Autodesk Fusion 360 part; units mm, degrees
(part 2 of 3)
sketch "Sketch22" plane through (0, -42.5, 42.5) normal (0, -0.707107, 0.707107) x (1, 0, 0) in component "BOX"
  line L0 (10.5, 0.9066) -> (16.8, 0.9066)
  line L1 (16.8, 0.9066) -> (16.8, -5.3934)
  line L2 (16.8, -5.3934) -> (10.5, -5.3934)
  line L3 (10.5, -5.3934) -> (10.5, -4.8934)
  line L4 (10.5, -4.8934) -> (16.5, -4.8934)
  line L5 (16.5, -4.8934) -> (16.5, 0.4066)
  line L6 (16.5, 0.4066) -> (10.5, 0.4066)
  line L7 (10.5, 0.4066) -> (10.5, 0.9066)
  line L8 (33.8, 0.9066) -> (40.1, 0.9066)
  line L9 (40.1, 0.9066) -> (40.1, -5.3934)
  line L10 (40.1, -5.3934) -> (33.8, -5.3934)
  line L11 (33.8, -5.3934) -> (33.8, -4.8934)
  line L12 (33.8, -4.8934) -> (39.8, -4.8934)
  line L13 (39.8, -4.8934) -> (39.8, 0.4066)
  line L14 (39.8, 0.4066) -> (33.8, 0.4066)
  line L15 (33.8, 0.4066) -> (33.8, 0.9066)
  line L16 (44.1, 0.9066) -> (50.4, 0.9066)
  line L17 (50.4, 0.9066) -> (50.4, -5.3934)
  line L18 (50.4, -5.3934) -> (44.1, -5.3934)
  line L19 (44.1, -5.3934) -> (44.1, -4.8934)
  line L20 (44.1, -4.8934) -> (50.1, -4.8934)
  line L21 (50.1, -4.8934) -> (50.1, 0.4066)
  line L22 (50.1, 0.4066) -> (44.1, 0.4066)
  line L23 (44.1, 0.4066) -> (44.1, 0.9066)
  line L24 (20.8, 0.9066) -> (27.1, 0.9066)
  line L25 (27.1, 0.9066) -> (27.1, -5.3934)
  line L26 (27.1, -5.3934) -> (20.8, -5.3934)
  line L27 (20.8, -5.3934) -> (20.8, -4.8934)
  line L28 (20.8, -4.8934) -> (26.8, -4.8934)
  line L29 (26.8, -4.8934) -> (26.8, 0.4066)
  line L30 (26.8, 0.4066) -> (20.8, 0.4066)
  line L31 (20.8, 0.4066) -> (20.8, 0.9066)
  line L32 (-10.3, 0.9066) -> (-4, 0.9066)
  line L33 (-4, 0.9066) -> (-4, -5.3934)
  line L34 (-4, -5.3934) -> (-10.3, -5.3934)
  line L35 (-10.3, -5.3934) -> (-10.3, -4.8934)
  line L36 (-10.3, -4.8934) -> (-4.3, -4.8934)
  line L37 (-4.3, -4.8934) -> (-4.3, 0.4066)
  line L38 (-4.3, 0.4066) -> (-10.3, 0.4066)
  line L39 (-10.3, 0.4066) -> (-10.3, 0.9066)
  line L40 (-54.5, -15.7434) -> (-54.5, 7.2566)
  line L41 (-54.5, 7.2566) -> (-20, 7.2566)
  line L42 (-20, 7.2566) -> (-20, -15.7434)
  line L43 (-20, -15.7434) -> (-54.5, -15.7434)
  line L44 (65, -24.7487) -> (65, 17.6777)
  line L45 (65, 17.6777) -> (-65, 17.6777)
  line L46 (-65, 17.6777) -> (-65, -24.7487)
  line L47 (-65, -24.7487) -> (65, -24.7487)
  line L48 (-10.546, -7.6932) -> (-10.2963, -7.6713)
  spline S0 degree 2 poles (-10.2963, -7.6713) (-10.2786, -7.8214) (-10.2138, -7.9176) knots 0 0 0 1 1 1
  spline S1 degree 2 poles (-10.2138, -7.9176) (-10.149, -8.0138) (-10.0125, -8.0731) knots 0 0 0 1 1 1
  spline S2 degree 2 poles (-10.0125, -8.0731) (-9.8761, -8.1325) (-9.7056, -8.1325) knots 0 0 0 1 1 1
  spline S3 degree 2 poles (-9.7056, -8.1325) (-9.5541, -8.1325) (-9.4382, -8.0874) knots 0 0 0 1 1 1
  spline S4 degree 2 poles (-9.4382, -8.0874) (-9.3222, -8.0424) (-9.2656, -7.964) knots 0 0 0 1 1 1
  spline S5 degree 2 poles (-9.2656, -7.964) (-9.209, -7.8855) (-9.209, -7.7928) knots 0 0 0 1 1 1
  spline S6 degree 2 poles (-9.209, -7.7928) (-9.209, -7.6986) (-9.2636, -7.6284) knots 0 0 0 1 1 1
  spline S7 degree 2 poles (-9.2636, -7.6284) (-9.3181, -7.5581) (-9.4436, -7.5104) knots 0 0 0 1 1 1
  spline S8 degree 2 poles (-9.4436, -7.5104) (-9.5241, -7.479) (-9.7997, -7.4128) knots 0 0 0 1 1 1
  spline S9 degree 2 poles (-9.7997, -7.4128) (-10.0753, -7.3467) (-10.1858, -7.288) knots 0 0 0 1 1 1
  spline S10 degree 2 poles (-10.1858, -7.288) (-10.329, -7.213) (-10.3993, -7.1018) knots 0 0 0 1 1 1
  spline S11 degree 2 poles (-10.3993, -7.1018) (-10.4696, -6.9906) (-10.4696, -6.8528) knots 0 0 0 1 1 1
  spline S12 degree 2 poles (-10.4696, -6.8528) (-10.4696, -6.7014) (-10.3836, -6.5697) knots 0 0 0 1 1 1
  spline S13 degree 2 poles (-10.3836, -6.5697) (-10.2977, -6.4381) (-10.1326, -6.3698) knots 0 0 0 1 1 1
  spline S14 degree 2 poles (-10.1326, -6.3698) (-9.9675, -6.3016) (-9.7656, -6.3016) knots 0 0 0 1 1 1
  spline S15 degree 2 poles (-9.7656, -6.3016) (-9.5432, -6.3016) (-9.3734, -6.3733) knots 0 0 0 1 1 1
  spline S16 degree 2 poles (-9.3734, -6.3733) (-9.2035, -6.4449) (-9.1121, -6.584) knots 0 0 0 1 1 1
  spline S17 degree 2 poles (-9.1121, -6.584) (-9.0207, -6.7232) (-9.0139, -6.8992) knots 0 0 0 1 1 1
  line L49 (-9.0139, -6.8992) -> (-9.2676, -6.9183)
  spline S18 degree 2 poles (-9.2676, -6.9183) (-9.2881, -6.7286) (-9.4061, -6.6318) knots 0 0 0 1 1 1
  spline S19 degree 2 poles (-9.4061, -6.6318) (-9.5241, -6.5349) (-9.7547, -6.5349) knots 0 0 0 1 1 1
  spline S20 degree 2 poles (-9.7547, -6.5349) (-9.9948, -6.5349) (-10.1046, -6.6229) knots 0 0 0 1 1 1
  spline S21 degree 2 poles (-10.1046, -6.6229) (-10.2144, -6.7109) (-10.2144, -6.8351) knots 0 0 0 1 1 1
  spline S22 degree 2 poles (-10.2144, -6.8351) (-10.2144, -6.9428) (-10.1367, -7.0124) knots 0 0 0 1 1 1
  spline S23 degree 2 poles (-10.1367, -7.0124) (-10.0603, -7.082) (-9.7376, -7.155) knots 0 0 0 1 1 1
  spline S24 degree 2 poles (-9.7376, -7.155) (-9.415, -7.228) (-9.2949, -7.2825) knots 0 0 0 1 1 1
  spline S25 degree 2 poles (-9.2949, -7.2825) (-9.1203, -7.363) (-9.0371, -7.4865) knots 0 0 0 1 1 1
  spline S26 degree 2 poles (-9.0371, -7.4865) (-8.9539, -7.61) (-8.9539, -7.7709) knots 0 0 0 1 1 1
  spline S27 degree 2 poles (-8.9539, -7.7709) (-8.9539, -7.9306) (-9.0453, -8.0718) knots 0 0 0 1 1 1
  spline S28 degree 2 poles (-9.0453, -8.0718) (-9.1367, -8.213) (-9.3079, -8.2914) knots 0 0 0 1 1 1
  spline S29 degree 2 poles (-9.3079, -8.2914) (-9.4791, -8.3698) (-9.6933, -8.3698) knots 0 0 0 1 1 1
  spline S30 degree 2 poles (-9.6933, -8.3698) (-9.9648, -8.3698) (-10.1483, -8.2907) knots 0 0 0 1 1 1
  spline S31 degree 2 poles (-10.1483, -8.2907) (-10.3318, -8.2116) (-10.4361, -8.0527) knots 0 0 0 1 1 1
  spline S32 degree 2 poles (-10.4361, -8.0527) (-10.5405, -7.8937) (-10.546, -7.6932) knots 0 0 0 1 1 1
  line L50 (-8.0835, -8.3357) -> (-8.0835, -6.5718)
  line L51 (-8.0835, -6.5718) -> (-8.7424, -6.5718)
  line L52 (-8.7424, -6.5718) -> (-8.7424, -6.3357)
  line L53 (-8.7424, -6.3357) -> (-7.1571, -6.3357)
  line L54 (-7.1571, -6.3357) -> (-7.1571, -6.5718)
  line L55 (-7.1571, -6.5718) -> (-7.8188, -6.5718)
  line L56 (-7.8188, -6.5718) -> (-7.8188, -8.3357)
  line L57 (-7.8188, -8.3357) -> (-8.0835, -8.3357)
  line L58 (-7.3127, -8.3357) -> (-6.5446, -6.3357)
  line L59 (-6.5446, -6.3357) -> (-6.2595, -6.3357)
  line L60 (-6.2595, -6.3357) -> (-5.4409, -8.3357)
  line L61 (-5.4409, -8.3357) -> (-5.7424, -8.3357)
  line L62 (-5.7424, -8.3357) -> (-5.9757, -7.73)
  line L63 (-5.9757, -7.73) -> (-6.812, -7.73)
  line L64 (-6.812, -7.73) -> (-7.0316, -8.3357)
  line L65 (-7.0316, -8.3357) -> (-7.3127, -8.3357)
  line L66 (-6.7356, -7.5145) -> (-6.0575, -7.5145)
  line L67 (-6.0575, -7.5145) -> (-6.2663, -6.9606)
  spline S33 degree 2 poles (-6.2663, -6.9606) (-6.3618, -6.7082) (-6.4082, -6.5458) knots 0 0 0 1 1 1
  spline S34 degree 2 poles (-6.4082, -6.5458) (-6.4464, -6.7382) (-6.5159, -6.9278) knots 0 0 0 1 1 1
  line L68 (-6.5159, -6.9278) -> (-6.7356, -7.5145)
  line L69 (-5.2254, -8.3357) -> (-5.2254, -6.3357)
  line L70 (-5.2254, -6.3357) -> (-4.3386, -6.3357)
  spline S35 degree 2 poles (-4.3386, -6.3357) (-4.0712, -6.3357) (-3.932, -6.3896) knots 0 0 0 1 1 1
  spline S36 degree 2 poles (-3.932, -6.3896) (-3.7929, -6.4435) (-3.7097, -6.5799) knots 0 0 0 1 1 1
  spline S37 degree 2 poles (-3.7097, -6.5799) (-3.6264, -6.7164) (-3.6264, -6.8814) knots 0 0 0 1 1 1
  spline S38 degree 2 poles (-3.6264, -6.8814) (-3.6264, -7.0943) (-3.7642, -7.2402) knots 0 0 0 1 1 1
  spline S39 degree 2 poles (-3.7642, -7.2402) (-3.902, -7.3862) (-4.1899, -7.4258) knots 0 0 0 1 1 1
  spline S40 degree 2 poles (-4.1899, -7.4258) (-4.0848, -7.4763) (-4.0303, -7.5254) knots 0 0 0 1 1 1
  spline S41 degree 2 poles (-4.0303, -7.5254) (-3.9143, -7.6318) (-3.8106, -7.7914) knots 0 0 0 1 1 1
  line L71 (-3.8106, -7.7914) -> (-3.4627, -8.3357)
  line L72 (-3.4627, -8.3357) -> (-3.7956, -8.3357)
  line L73 (-3.7956, -8.3357) -> (-4.0603, -7.9196)
  spline S42 degree 2 poles (-4.0603, -7.9196) (-4.1762, -7.7396) (-4.2513, -7.6441) knots 0 0 0 1 1 1
  spline S43 degree 2 poles (-4.2513, -7.6441) (-4.3263, -7.5486) (-4.3857, -7.5104) knots 0 0 0 1 1 1
  spline S44 degree 2 poles (-4.3857, -7.5104) (-4.445, -7.4722) (-4.5064, -7.4572) knots 0 0 0 1 1 1
  spline S45 degree 2 poles (-4.5064, -7.4572) (-4.5514, -7.4476) (-4.6537, -7.4476) knots 0 0 0 1 1 1
  line L74 (-4.6537, -7.4476) -> (-4.9607, -7.4476)
  line L75 (-4.9607, -7.4476) -> (-4.9607, -8.3357)
  line L76 (-4.9607, -8.3357) -> (-5.2254, -8.3357)
  line L77 (-4.9607, -7.2184) -> (-4.3918, -7.2184)
  spline S46 degree 2 poles (-4.3918, -7.2184) (-4.2103, -7.2184) (-4.108, -7.1809) knots 0 0 0 1 1 1
  spline S47 degree 2 poles (-4.108, -7.1809) (-4.0057, -7.1434) (-3.9525, -7.0608) knots 0 0 0 1 1 1
  spline S48 degree 2 poles (-3.9525, -7.0608) (-3.8993, -6.9783) (-3.8993, -6.8814) knots 0 0 0 1 1 1
  spline S49 degree 2 poles (-3.8993, -6.8814) (-3.8993, -6.7396) (-4.0023, -6.6482) knots 0 0 0 1 1 1
  spline S50 degree 2 poles (-4.0023, -6.6482) (-4.1053, -6.5567) (-4.3277, -6.5567) knots 0 0 0 1 1 1
  line L78 (-4.3277, -6.5567) -> (-4.9607, -6.5567)
  line L79 (-4.9607, -6.5567) -> (-4.9607, -7.2184)
  line L80 (-2.7533, -8.3357) -> (-2.7533, -6.5718)
  line L81 (-2.7533, -6.5718) -> (-3.4123, -6.5718)
  line L82 (-3.4123, -6.5718) -> (-3.4123, -6.3357)
  line L83 (-3.4123, -6.3357) -> (-1.827, -6.3357)
  line L84 (-1.827, -6.3357) -> (-1.827, -6.5718)
  line L85 (-1.827, -6.5718) -> (-2.4887, -6.5718)
  line L86 (-2.4887, -6.5718) -> (-2.4887, -8.3357)
  line L87 (-2.4887, -8.3357) -> (-2.7533, -8.3357)
  line L88 (-9.7656, -6.3016) -> (65, -6.3016) construction
  line L89 (10.1816, -8.2989) -> (10.1816, -6.2989)
  line L90 (10.1816, -6.2989) -> (10.58, -6.2989)
  line L91 (10.58, -6.2989) -> (11.0533, -7.715)
  spline S51 degree 2 poles (11.0533, -7.715) (11.1188, -7.9129) (11.1488, -8.0111) knots 0 0 0 1 1 1
  spline S52 degree 2 poles (11.1488, -8.0111) (11.183, -7.9019) (11.2553, -7.6905) knots 0 0 0 1 1 1
  line L92 (11.2553, -7.6905) -> (11.7341, -6.2989)
  line L93 (11.7341, -6.2989) -> (12.0902, -6.2989)
  line L94 (12.0902, -6.2989) -> (12.0902, -8.2989)
  line L95 (12.0902, -8.2989) -> (11.8351, -8.2989)
  line L96 (11.8351, -8.2989) -> (11.8351, -6.625)
  line L97 (11.8351, -6.625) -> (11.2539, -8.2989)
  line L98 (11.2539, -8.2989) -> (11.0151, -8.2989)
  line L99 (11.0151, -8.2989) -> (10.4367, -6.5963)
  line L100 (10.4367, -6.5963) -> (10.4367, -8.2989)
  line L101 (10.4367, -8.2989) -> (10.1816, -8.2989)
  line L102 (12.5227, -8.2989) -> (12.5227, -6.2989)
  line L103 (12.5227, -6.2989) -> (13.9688, -6.2989)
  line L104 (13.9688, -6.2989) -> (13.9688, -6.535)
  line L105 (13.9688, -6.535) -> (12.7873, -6.535)
  line L106 (12.7873, -6.535) -> (12.7873, -7.1475)
  line L107 (12.7873, -7.1475) -> (13.8937, -7.1475)
  line L108 (13.8937, -7.1475) -> (13.8937, -7.3822)
  line L109 (13.8937, -7.3822) -> (12.7873, -7.3822)
  line L110 (12.7873, -7.3822) -> (12.7873, -8.0629)
  line L111 (12.7873, -8.0629) -> (14.0151, -8.0629)
  line L112 (14.0151, -8.0629) -> (14.0151, -8.2989)
  line L113 (14.0151, -8.2989) -> (12.5227, -8.2989)
  line L114 (14.378, -8.2989) -> (14.378, -6.2989)
  line L115 (14.378, -6.2989) -> (14.6495, -6.2989)
  line L116 (14.6495, -6.2989) -> (15.7, -7.8692)
  line L117 (15.7, -7.8692) -> (15.7, -6.2989)
  line L118 (15.7, -6.2989) -> (15.9538, -6.2989)
  line L119 (15.9538, -6.2989) -> (15.9538, -8.2989)
  line L120 (15.9538, -8.2989) -> (15.6823, -8.2989)
  line L121 (15.6823, -8.2989) -> (14.6318, -6.7273)
  line L122 (14.6318, -6.7273) -> (14.6318, -8.2989)
  line L123 (14.6318, -8.2989) -> (14.378, -8.2989)
  line L124 (17.7109, -6.2989) -> (17.9756, -6.2989)
  line L125 (17.9756, -6.2989) -> (17.9756, -7.4545)
  spline S53 degree 2 poles (17.9756, -7.4545) (17.9756, -7.756) (17.9074, -7.9333) knots 0 0 0 1 1 1
  spline S54 degree 2 poles (17.9074, -7.9333) (17.8392, -8.1107) (17.6611, -8.2219) knots 0 0 0 1 1 1
  spline S55 degree 2 poles (17.6611, -8.2219) (17.4831, -8.333) (17.1939, -8.333) knots 0 0 0 1 1 1
  spline S56 degree 2 poles (17.1939, -8.333) (16.9128, -8.333) (16.7341, -8.2362) knots 0 0 0 1 1 1
  spline S57 degree 2 poles (16.7341, -8.2362) (16.5554, -8.1393) (16.479, -7.9558) knots 0 0 0 1 1 1
  spline S58 degree 2 poles (16.479, -7.9558) (16.4026, -7.7723) (16.4026, -7.4545) knots 0 0 0 1 1 1
  line L126 (16.4026, -7.4545) -> (16.4026, -6.2989)
  line L127 (16.4026, -6.2989) -> (16.6673, -6.2989)
  line L128 (16.6673, -6.2989) -> (16.6673, -7.4531)
  spline S59 degree 2 poles (16.6673, -7.4531) (16.6673, -7.7137) (16.7157, -7.8371) knots 0 0 0 1 1 1
  spline S60 degree 2 poles (16.7157, -7.8371) (16.7641, -7.9606) (16.8821, -8.0274) knots 0 0 0 1 1 1
  spline S61 degree 2 poles (16.8821, -8.0274) (17.0001, -8.0943) (17.1707, -8.0943) knots 0 0 0 1 1 1
  spline S62 degree 2 poles (17.1707, -8.0943) (17.4626, -8.0943) (17.5868, -7.962) knots 0 0 0 1 1 1
  spline S63 degree 2 poles (17.5868, -7.962) (17.7109, -7.8296) (17.7109, -7.4531) knots 0 0 0 1 1 1
  line L129 (17.7109, -7.4531) -> (17.7109, -6.2989)
  line L130 (20.4857, -7.8167) -> (20.7354, -7.7948)
  spline S64 degree 2 poles (20.7354, -7.7948) (20.7531, -7.9449) (20.8179, -8.0411) knots 0 0 0 1 1 1
  spline S65 degree 2 poles (20.8179, -8.0411) (20.8827, -8.1373) (21.0191, -8.1966) knots 0 0 0 1 1 1
  spline S66 degree 2 poles (21.0191, -8.1966) (21.1556, -8.256) (21.3261, -8.256) knots 0 0 0 1 1 1
  spline S67 degree 2 poles (21.3261, -8.256) (21.4775, -8.256) (21.5935, -8.2109) knots 0 0 0 1 1 1
  spline S68 degree 2 poles (21.5935, -8.2109) (21.7094, -8.1659) (21.7661, -8.0875) knots 0 0 0 1 1 1
  spline S69 degree 2 poles (21.7661, -8.0875) (21.8227, -8.009) (21.8227, -7.9163) knots 0 0 0 1 1 1
  spline S70 degree 2 poles (21.8227, -7.9163) (21.8227, -7.8221) (21.7681, -7.7519) knots 0 0 0 1 1 1
  spline S71 degree 2 poles (21.7681, -7.7519) (21.7135, -7.6816) (21.588, -7.6339) knots 0 0 0 1 1 1
  spline S72 degree 2 poles (21.588, -7.6339) (21.5075, -7.6025) (21.2319, -7.5363) knots 0 0 0 1 1 1
  spline S73 degree 2 poles (21.2319, -7.5363) (20.9564, -7.4701) (20.8459, -7.4115) knots 0 0 0 1 1 1
  spline S74 degree 2 poles (20.8459, -7.4115) (20.7026, -7.3364) (20.6324, -7.2253) knots 0 0 0 1 1 1
  spline S75 degree 2 poles (20.6324, -7.2253) (20.5621, -7.1141) (20.5621, -6.9763) knots 0 0 0 1 1 1
  spline S76 degree 2 poles (20.5621, -6.9763) (20.5621, -6.8248) (20.648, -6.6932) knots 0 0 0 1 1 1
  spline S77 degree 2 poles (20.648, -6.6932) (20.734, -6.5615) (20.8991, -6.4933) knots 0 0 0 1 1 1
  spline S78 degree 2 poles (20.8991, -6.4933) (21.0641, -6.4251) (21.2661, -6.4251) knots 0 0 0 1 1 1
  spline S79 degree 2 poles (21.2661, -6.4251) (21.4884, -6.4251) (21.6583, -6.4967) knots 0 0 0 1 1 1
  spline S80 degree 2 poles (21.6583, -6.4967) (21.8281, -6.5684) (21.9195, -6.7075) knots 0 0 0 1 1 1
  spline S81 degree 2 poles (21.9195, -6.7075) (22.0109, -6.8467) (22.0178, -7.0227) knots 0 0 0 1 1 1
  line L131 (22.0178, -7.0227) -> (21.764, -7.0418)
  spline S82 degree 2 poles (21.764, -7.0418) (21.7435, -6.8521) (21.6255, -6.7553) knots 0 0 0 1 1 1
  spline S83 degree 2 poles (21.6255, -6.7553) (21.5075, -6.6584) (21.277, -6.6584) knots 0 0 0 1 1 1
  spline S84 degree 2 poles (21.277, -6.6584) (21.0369, -6.6584) (20.927, -6.7464) knots 0 0 0 1 1 1
  spline S85 degree 2 poles (20.927, -6.7464) (20.8172, -6.8344) (20.8172, -6.9585) knots 0 0 0 1 1 1
  spline S86 degree 2 poles (20.8172, -6.9585) (20.8172, -7.0663) (20.895, -7.1359) knots 0 0 0 1 1 1
  spline S87 degree 2 poles (20.895, -7.1359) (20.9714, -7.2055) (21.294, -7.2785) knots 0 0 0 1 1 1
  spline S88 degree 2 poles (21.294, -7.2785) (21.6167, -7.3514) (21.7367, -7.406) knots 0 0 0 1 1 1
  spline S89 degree 2 poles (21.7367, -7.406) (21.9113, -7.4865) (21.9946, -7.61) knots 0 0 0 1 1 1
  spline S90 degree 2 poles (21.9946, -7.61) (22.0778, -7.7334) (22.0778, -7.8944) knots 0 0 0 1 1 1
  spline S91 degree 2 poles (22.0778, -7.8944) (22.0778, -8.054) (21.9864, -8.1952) knots 0 0 0 1 1 1
  spline S92 degree 2 poles (21.9864, -8.1952) (21.895, -8.3364) (21.7238, -8.4149) knots 0 0 0 1 1 1
  spline S93 degree 2 poles (21.7238, -8.4149) (21.5525, -8.4933) (21.3384, -8.4933) knots 0 0 0 1 1 1
  spline S94 degree 2 poles (21.3384, -8.4933) (21.0669, -8.4933) (20.8834, -8.4142) knots 0 0 0 1 1 1
  spline S95 degree 2 poles (20.8834, -8.4142) (20.6999, -8.3351) (20.5955, -8.1761) knots 0 0 0 1 1 1
  spline S96 degree 2 poles (20.5955, -8.1761) (20.4912, -8.0172) (20.4857, -7.8167) knots 0 0 0 1 1 1
  line L132 (22.4448, -8.4592) -> (22.4448, -6.4592)
  line L133 (22.4448, -6.4592) -> (23.8909, -6.4592)
  line L134 (23.8909, -6.4592) -> (23.8909, -6.6952)
  line L135 (23.8909, -6.6952) -> (22.7094, -6.6952)
  line L136 (22.7094, -6.6952) -> (22.7094, -7.3078)
  line L137 (22.7094, -7.3078) -> (23.8159, -7.3078)
  line L138 (23.8159, -7.3078) -> (23.8159, -7.5424)
  line L139 (23.8159, -7.5424) -> (22.7094, -7.5424)
  line L140 (22.7094, -7.5424) -> (22.7094, -8.2232)
  line L141 (22.7094, -8.2232) -> (23.9373, -8.2232)
  line L142 (23.9373, -8.2232) -> (23.9373, -8.4592)
  line L143 (23.9373, -8.4592) -> (22.4448, -8.4592)
  line L144 (24.292, -8.4592) -> (24.292, -6.4592)
  line L145 (24.292, -6.4592) -> (24.5566, -6.4592)
  line L146 (24.5566, -6.4592) -> (24.5566, -8.2232)
  line L147 (24.5566, -8.2232) -> (25.5416, -8.2232)
  line L148 (25.5416, -8.2232) -> (25.5416, -8.4592)
  line L149 (25.5416, -8.4592) -> (24.292, -8.4592)
  line L150 (25.8622, -8.4592) -> (25.8622, -6.4592)
  line L151 (25.8622, -6.4592) -> (27.3083, -6.4592)
  line L152 (27.3083, -6.4592) -> (27.3083, -6.6952)
  line L153 (27.3083, -6.6952) -> (26.1269, -6.6952)
  line L154 (26.1269, -6.6952) -> (26.1269, -7.3078)
  line L155 (26.1269, -7.3078) -> (27.2333, -7.3078)
  line L156 (27.2333, -7.3078) -> (27.2333, -7.5424)
  line L157 (27.2333, -7.5424) -> (26.1269, -7.5424)
  line L158 (26.1269, -7.5424) -> (26.1269, -8.2232)
  line L159 (26.1269, -8.2232) -> (27.3547, -8.2232)
  line L160 (27.3547, -8.2232) -> (27.3547, -8.4592)
  line L161 (27.3547, -8.4592) -> (25.8622, -8.4592)
  line L162 (29.1474, -7.758) -> (29.412, -7.8248)
  spline S97 degree 2 poles (29.412, -7.8248) (29.3288, -8.1509) (29.1126, -8.3221) knots 0 0 0 1 1 1
  spline S98 degree 2 poles (29.1126, -8.3221) (28.8963, -8.4933) (28.5839, -8.4933) knots 0 0 0 1 1 1
  spline S99 degree 2 poles (28.5839, -8.4933) (28.2606, -8.4933) (28.058, -8.3617) knots 0 0 0 1 1 1
  spline S100 degree 2 poles (28.058, -8.3617) (27.8554, -8.23) (27.7497, -7.9804) knots 0 0 0 1 1 1
  spline S101 degree 2 poles (27.7497, -7.9804) (27.644, -7.7307) (27.644, -7.4442) knots 0 0 0 1 1 1
  spline S102 degree 2 poles (27.644, -7.4442) (27.644, -7.1318) (27.7633, -6.8992) knots 0 0 0 1 1 1
  spline S103 degree 2 poles (27.7633, -6.8992) (27.8827, -6.6666) (28.103, -6.5459) knots 0 0 0 1 1 1
  spline S104 degree 2 poles (28.103, -6.5459) (28.3234, -6.4251) (28.588, -6.4251) knots 0 0 0 1 1 1
  spline S105 degree 2 poles (28.588, -6.4251) (28.8882, -6.4251) (29.0928, -6.5779) knots 0 0 0 1 1 1
  spline S106 degree 2 poles (29.0928, -6.5779) (29.2974, -6.7307) (29.3779, -7.0077) knots 0 0 0 1 1 1
  line L163 (29.3779, -7.0077) -> (29.1174, -7.069)
  spline S107 degree 2 poles (29.1174, -7.069) (29.0478, -6.8508) (28.9154, -6.7512) knots 0 0 0 1 1 1
  spline S108 degree 2 poles (28.9154, -6.7512) (28.7831, -6.6516) (28.5826, -6.6516) knots 0 0 0 1 1 1
  spline S109 degree 2 poles (28.5826, -6.6516) (28.352, -6.6516) (28.1972, -6.7621) knots 0 0 0 1 1 1
  spline S110 degree 2 poles (28.1972, -6.7621) (28.0423, -6.8726) (27.9796, -7.0588) knots 0 0 0 1 1 1
  spline S111 degree 2 poles (27.9796, -7.0588) (27.9168, -7.245) (27.9168, -7.4429) knots 0 0 0 1 1 1
  spline S112 degree 2 poles (27.9168, -7.4429) (27.9168, -7.698) (27.9912, -7.8883) knots 0 0 0 1 1 1
  spline S113 degree 2 poles (27.9912, -7.8883) (28.0655, -8.0786) (28.2224, -8.1727) knots 0 0 0 1 1 1
  spline S114 degree 2 poles (28.2224, -8.1727) (28.3793, -8.2669) (28.5621, -8.2669) knots 0 0 0 1 1 1
  spline S115 degree 2 poles (28.5621, -8.2669) (28.7845, -8.2669) (28.9386, -8.1386) knots 0 0 0 1 1 1
  spline S116 degree 2 poles (28.9386, -8.1386) (29.0928, -8.0104) (29.1474, -7.758) knots 0 0 0 1 1 1
  line L164 (30.247, -8.4592) -> (30.247, -6.6952)
  line L165 (30.247, -6.6952) -> (29.588, -6.6952)
  line L166 (29.588, -6.6952) -> (29.588, -6.4592)
  line L167 (29.588, -6.4592) -> (31.1733, -6.4592)
  line L168 (31.1733, -6.4592) -> (31.1733, -6.6952)
  line L169 (31.1733, -6.6952) -> (30.5116, -6.6952)
  line L170 (30.5116, -6.6952) -> (30.5116, -8.4592)
  line L171 (30.5116, -8.4592) -> (30.247, -8.4592)
  line L172 (36.1107, -6.5124) -> (36.3754, -6.5124)
  line L173 (36.3754, -6.5124) -> (36.3754, -7.668)
  spline S117 degree 2 poles (36.3754, -7.668) (36.3754, -7.9695) (36.3072, -8.1468) knots 0 0 0 1 1 1
  spline S118 degree 2 poles (36.3072, -8.1468) (36.2389, -8.3242) (36.0609, -8.4354) knots 0 0 0 1 1 1
  spline S119 degree 2 poles (36.0609, -8.4354) (35.8829, -8.5465) (35.5936, -8.5465) knots 0 0 0 1 1 1
  spline S120 degree 2 poles (35.5936, -8.5465) (35.3126, -8.5465) (35.1339, -8.4497) knots 0 0 0 1 1 1
  spline S121 degree 2 poles (35.1339, -8.4497) (34.9552, -8.3528) (34.8788, -8.1693) knots 0 0 0 1 1 1
  spline S122 degree 2 poles (34.8788, -8.1693) (34.8024, -7.9858) (34.8024, -7.668) knots 0 0 0 1 1 1
  line L174 (34.8024, -7.668) -> (34.8024, -6.5124)
  line L175 (34.8024, -6.5124) -> (35.067, -6.5124)
  line L176 (35.067, -6.5124) -> (35.067, -7.6666)
  spline S123 degree 2 poles (35.067, -7.6666) (35.067, -7.9272) (35.1155, -8.0506) knots 0 0 0 1 1 1
  spline S124 degree 2 poles (35.1155, -8.0506) (35.1639, -8.1741) (35.2819, -8.2409) knots 0 0 0 1 1 1
  spline S125 degree 2 poles (35.2819, -8.2409) (35.3999, -8.3078) (35.5705, -8.3078) knots 0 0 0 1 1 1
  spline S126 degree 2 poles (35.5705, -8.3078) (35.8624, -8.3078) (35.9866, -8.1755) knots 0 0 0 1 1 1
  spline S127 degree 2 poles (35.9866, -8.1755) (36.1107, -8.0431) (36.1107, -7.6666) knots 0 0 0 1 1 1
  line L177 (36.1107, -7.6666) -> (36.1107, -6.5124)
  line L178 (36.816, -8.5124) -> (36.816, -6.5124)
  line L179 (36.816, -6.5124) -> (37.5705, -6.5124)
  spline S128 degree 2 poles (37.5705, -6.5124) (37.7696, -6.5124) (37.8747, -6.5315) knots 0 0 0 1 1 1
  spline S129 degree 2 poles (37.8747, -6.5315) (38.022, -6.5561) (38.1216, -6.625) knots 0 0 0 1 1 1
  spline S130 degree 2 poles (38.1216, -6.625) (38.2212, -6.6939) (38.2819, -6.818) knots 0 0 0 1 1 1
  spline S131 degree 2 poles (38.2819, -6.818) (38.3426, -6.9422) (38.3426, -7.0909) knots 0 0 0 1 1 1
  spline S132 degree 2 poles (38.3426, -7.0909) (38.3426, -7.346) (38.1803, -7.5227) knots 0 0 0 1 1 1
  spline S133 degree 2 poles (38.1803, -7.5227) (38.0179, -7.6993) (37.5936, -7.6993) knots 0 0 0 1 1 1
  line L180 (37.5936, -7.6993) -> (37.0807, -7.6993)
  line L181 (37.0807, -7.6993) -> (37.0807, -8.5124)
  line L182 (37.0807, -8.5124) -> (36.816, -8.5124)
  line L183 (37.0807, -7.4633) -> (37.5977, -7.4633)
  spline S134 degree 2 poles (37.5977, -7.4633) (37.8542, -7.4633) (37.962, -7.3678) knots 0 0 0 1 1 1
  spline S135 degree 2 poles (37.962, -7.3678) (38.0698, -7.2723) (38.0698, -7.0991) knots 0 0 0 1 1 1
  spline S136 degree 2 poles (38.0698, -7.0991) (38.0698, -6.9736) (38.0063, -6.8842) knots 0 0 0 1 1 1
  spline S137 degree 2 poles (38.0063, -6.8842) (37.9429, -6.7948) (37.8392, -6.7662) knots 0 0 0 1 1 1
  spline S138 degree 2 poles (37.8392, -6.7662) (37.7724, -6.7485) (37.5923, -6.7485) knots 0 0 0 1 1 1
  line L184 (37.5923, -6.7485) -> (37.0807, -6.7485)
  line L185 (37.0807, -6.7485) -> (37.0807, -7.4633)
  line L186 (38.464, -8.5465) -> (39.0439, -6.4783)
  line L187 (39.0439, -6.4783) -> (39.2403, -6.4783)
  line L188 (39.2403, -6.4783) -> (38.6619, -8.5465)
  line L189 (38.6619, -8.5465) -> (38.464, -8.5465)
  line L190 (39.9402, -8.1891) -> (39.9402, -7.6407)
  line L191 (39.9402, -7.6407) -> (39.3958, -7.6407)
  line L192 (39.3958, -7.6407) -> (39.3958, -7.4115)
  line L193 (39.3958, -7.4115) -> (39.9402, -7.4115)
  line L194 (39.9402, -7.4115) -> (39.9402, -6.8671)
  line L195 (39.9402, -6.8671) -> (40.1721, -6.8671)
  line L196 (40.1721, -6.8671) -> (40.1721, -7.4115)
  line L197 (40.1721, -7.4115) -> (40.7164, -7.4115)
  line L198 (40.7164, -7.4115) -> (40.7164, -7.6407)
  line L199 (40.7164, -7.6407) -> (40.1721, -7.6407)
  line L200 (40.1721, -7.6407) -> (40.1721, -8.1891)
  line L201 (40.1721, -8.1891) -> (39.9402, -8.1891)
  line L202 (43.102, -8.34) -> (43.102, -6.34)
  line L203 (43.102, -6.34) -> (43.7909, -6.34)
  spline S139 degree 2 poles (43.7909, -6.34) (44.0242, -6.34) (44.147, -6.3686) knots 0 0 0 1 1 1
  spline S140 degree 2 poles (44.147, -6.3686) (44.3189, -6.4082) (44.4403, -6.5119) knots 0 0 0 1 1 1
  spline S141 degree 2 poles (44.4403, -6.5119) (44.5985, -6.6456) (44.677, -6.8536) knots 0 0 0 1 1 1
  spline S142 degree 2 poles (44.677, -6.8536) (44.7554, -7.0617) (44.7554, -7.3291) knots 0 0 0 1 1 1
  spline S143 degree 2 poles (44.7554, -7.3291) (44.7554, -7.5569) (44.7022, -7.7329) knots 0 0 0 1 1 1
  spline S144 degree 2 poles (44.7022, -7.7329) (44.649, -7.9089) (44.5658, -8.0242) knots 0 0 0 1 1 1
  spline S145 degree 2 poles (44.5658, -8.0242) (44.4826, -8.1394) (44.3837, -8.2056) knots 0 0 0 1 1 1
  spline S146 degree 2 poles (44.3837, -8.2056) (44.2848, -8.2718) (44.1449, -8.3059) knots 0 0 0 1 1 1
  spline S147 degree 2 poles (44.1449, -8.3059) (44.0051, -8.34) (43.8237, -8.34) knots 0 0 0 1 1 1
  line L204 (43.8237, -8.34) -> (43.102, -8.34)
  line L205 (43.3666, -8.104) -> (43.7936, -8.104)
  spline S148 degree 2 poles (43.7936, -8.104) (43.9915, -8.104) (44.104, -8.0671) knots 0 0 0 1 1 1
  spline S149 degree 2 poles (44.104, -8.0671) (44.2166, -8.0303) (44.2834, -7.9635) knots 0 0 0 1 1 1
  spline S150 degree 2 poles (44.2834, -7.9635) (44.3775, -7.8693) (44.4301, -7.7104) knots 0 0 0 1 1 1
  spline S151 degree 2 poles (44.4301, -7.7104) (44.4826, -7.5515) (44.4826, -7.325) knots 0 0 0 1 1 1
  spline S152 degree 2 poles (44.4826, -7.325) (44.4826, -7.0112) (44.3796, -6.8427) knots 0 0 0 1 1 1
  spline S153 degree 2 poles (44.3796, -6.8427) (44.2766, -6.6742) (44.1292, -6.6169) knots 0 0 0 1 1 1
  spline S154 degree 2 poles (44.1292, -6.6169) (44.0228, -6.576) (43.7868, -6.576) knots 0 0 0 1 1 1
  line L206 (43.7868, -6.576) -> (43.3666, -6.576)
  line L207 (43.3666, -6.576) -> (43.3666, -8.104)
  spline S155 degree 2 poles (45.0392, -7.3659) (45.0392, -6.868) (45.3066, -6.5862) knots 0 0 0 1 1 1
  spline S156 degree 2 poles (45.3066, -6.5862) (45.574, -6.3045) (45.9969, -6.3045) knots 0 0 0 1 1 1
  spline S157 degree 2 poles (45.9969, -6.3045) (46.2739, -6.3045) (46.4962, -6.4369) knots 0 0 0 1 1 1
  spline S158 degree 2 poles (46.4962, -6.4369) (46.7186, -6.5692) (46.8352, -6.8059) knots 0 0 0 1 1 1
  spline S159 degree 2 poles (46.8352, -6.8059) (46.9519, -7.0426) (46.9519, -7.3427) knots 0 0 0 1 1 1
  spline S160 degree 2 poles (46.9519, -7.3427) (46.9519, -7.6469) (46.8291, -7.8871) knots 0 0 0 1 1 1
  spline S161 degree 2 poles (46.8291, -7.8871) (46.7063, -8.1272) (46.4812, -8.2506) knots 0 0 0 1 1 1
  spline S162 degree 2 poles (46.4812, -8.2506) (46.2561, -8.3741) (45.9955, -8.3741) knots 0 0 0 1 1 1
  spline S163 degree 2 poles (45.9955, -8.3741) (45.7131, -8.3741) (45.4908, -8.2377) knots 0 0 0 1 1 1
  spline S164 degree 2 poles (45.4908, -8.2377) (45.2684, -8.1012) (45.1538, -7.8652) knots 0 0 0 1 1 1
  spline S165 degree 2 poles (45.1538, -7.8652) (45.0392, -7.6292) (45.0392, -7.3659) knots 0 0 0 1 1 1
  spline S166 degree 2 poles (45.3121, -7.37) (45.3121, -7.7315) (45.5065, -7.9396) knots 0 0 0 1 1 1
  spline S167 degree 2 poles (45.5065, -7.9396) (45.7009, -8.1476) (45.9942, -8.1476) knots 0 0 0 1 1 1
  spline S168 degree 2 poles (45.9942, -8.1476) (46.293, -8.1476) (46.486, -7.9375) knots 0 0 0 1 1 1
  spline S169 degree 2 poles (46.486, -7.9375) (46.679, -7.7274) (46.679, -7.3414) knots 0 0 0 1 1 1
  spline S170 degree 2 poles (46.679, -7.3414) (46.679, -7.0972) (46.5965, -6.915) knots 0 0 0 1 1 1
  spline S171 degree 2 poles (46.5965, -6.915) (46.514, -6.7329) (46.355, -6.6326) knots 0 0 0 1 1 1
  spline S172 degree 2 poles (46.355, -6.6326) (46.1961, -6.5324) (45.9983, -6.5324) knots 0 0 0 1 1 1
  spline S173 degree 2 poles (45.9983, -6.5324) (45.7172, -6.5324) (45.5146, -6.7254) knots 0 0 0 1 1 1
  spline S174 degree 2 poles (45.5146, -6.7254) (45.3121, -6.9184) (45.3121, -7.37) knots 0 0 0 1 1 1
  line L208 (47.6422, -8.34) -> (47.1115, -6.34)
  line L209 (47.1115, -6.34) -> (47.383, -6.34)
  line L210 (47.383, -6.34) -> (47.6872, -7.651)
  spline S175 degree 2 poles (47.6872, -7.651) (47.7363, -7.857) (47.7718, -8.0603) knots 0 0 0 1 1 1
  spline S176 degree 2 poles (47.7718, -8.0603) (47.8482, -7.7397) (47.8618, -7.6906) knots 0 0 0 1 1 1
  line L211 (47.8618, -7.6906) -> (48.2425, -6.34)
  line L212 (48.2425, -6.34) -> (48.5617, -6.34)
  line L213 (48.5617, -6.34) -> (48.8482, -7.3523)
  spline S177 degree 2 poles (48.8482, -7.3523) (48.956, -7.7288) (49.0037, -8.0603) knots 0 0 0 1 1 1
  spline S178 degree 2 poles (49.0037, -8.0603) (49.0419, -7.8707) (49.1033, -7.6251) knots 0 0 0 1 1 1
  line L214 (49.1033, -7.6251) -> (49.4171, -6.34)
  line L215 (49.4171, -6.34) -> (49.6831, -6.34)
  line L216 (49.6831, -6.34) -> (49.1347, -8.34)
  line L217 (49.1347, -8.34) -> (48.8796, -8.34)
  line L218 (48.8796, -8.34) -> (48.458, -6.8161)
  spline S179 degree 2 poles (48.458, -6.8161) (48.4048, -6.6251) (48.3953, -6.5815) knots 0 0 0 1 1 1
  spline S180 degree 2 poles (48.3953, -6.5815) (48.3639, -6.7193) (48.3366, -6.8161) knots 0 0 0 1 1 1
  line L219 (48.3366, -6.8161) -> (47.9123, -8.34)
  line L220 (47.9123, -8.34) -> (47.6422, -8.34)
  line L221 (49.9273, -8.34) -> (49.9273, -6.34)
  line L222 (49.9273, -6.34) -> (50.1988, -6.34)
  line L223 (50.1988, -6.34) -> (51.2493, -7.9102)
  line L224 (51.2493, -7.9102) -> (51.2493, -6.34)
  line L225 (51.2493, -6.34) -> (51.503, -6.34)
  line L226 (51.503, -6.34) -> (51.503, -8.34)
  line L227 (51.503, -8.34) -> (51.2316, -8.34)
  line L228 (51.2316, -8.34) -> (50.1811, -6.7684)
  line L229 (50.1811, -6.7684) -> (50.1811, -8.34)
  line L230 (50.1811, -8.34) -> (49.9273, -8.34)
  line L231 (51.7322, -8.3741) -> (52.3121, -6.3059)
  line L232 (52.3121, -6.3059) -> (52.5085, -6.3059)
  line L233 (52.5085, -6.3059) -> (51.9301, -8.3741)
  line L234 (51.9301, -8.3741) -> (51.7322, -8.3741)
  line L235 (52.5972, -7.7397) -> (52.5972, -7.4928)
  line L236 (52.5972, -7.4928) -> (53.3516, -7.4928)
  line L237 (53.3516, -7.4928) -> (53.3516, -7.7397)
  line L238 (53.3516, -7.7397) -> (52.5972, -7.7397)
  constraint coincident L44 L88.end
extrude "Extrude23" cut sketch "Sketch22" against normal blind 3 contours L48 S0 S1 S2 S3 S4 S5 S6 S7 S8 S9 S10 S11 S12 S13 S14 S15 S16 S17 L49 S18 S19 S20 S21 S22 S23 S24 S25 S26 S27 S28 S29 S30 S31 S32 | L50 L51 L52 L53 L54 L55 L56 L57 | L58 L59 L60 L61 L62 L63 L64 L65 | L69 L70 S35 S36 S37 S38 S39 S40 S41 L71 L72 L73 S42 S43 S44 S45 L74 L75 L76 | L80 L81 L82 L83 L84 L85 L86 L87 | L89 L90 L91 S51 S52 L92 L93 L94 L95 L96 L97 L98 L99 L100 L101 | L102 L103 L104 L105 L106 L107 L108 L109 L110 L111 L112 L113 | L114 L115 L116 L117 L118 L119 L120 L121 L122 L123 | L124 L125 S53 S54 S55 S56 S57 S58 L126 L127 L128 S59 S60 S61 S62 S63 L129 | L130 S64 S65 S66 S67 S68 S69 S70 S71 S72 S73 S74 S75 S76 S77 S78 S79 S80 S81 L131 S82 S83 S84 S85 S86 S87 S88 S89 S90 S91 S92 S93 S94 S95 S96 | L132 L133 L134 L135 L136 L137 L138 L139 L140 L141 L142 L143 | L144 L145 L146 L147 L148 L149 | L150 L151 L152 L153 L154 L155 L156 L157 L158 L159 L160 L161 | L162 S97 S98 S99 S100 S101 S102 S103 S104 S105 S106 L163 S107 S108 S109 S110 S111 S112 S113 S114 S115 S116 | L164 L165 L166 L167 L168 L169 L170 L171 | L172 L173 S117 S118 S119 S120 S121 S122 L174 L175 L176 S123 S124 S125 S126 S127 L177 | L178 L179 S128 S129 S130 S131 S132 S133 L180 L181 L182 | L186 L187 L188 L189 | L190 L191 L192 L193 L194 L195 L196 L197 L198 L199 L200 L201 | L202 L203 S139 S140 S141 S142 S143 S144 S145 S146 S147 L204 | S155 S156 S157 S158 S159 S160 S161 S162 S163 S164 S165 | L208 L209 L210 S175 S176 L211 L212 L213 S177 S178 L214 L215 L216 L217 L218 S179 S180 L219 L220 | L221 L222 L223 L224 L225 L226 L227 L228 L229 L230 | L231 L232 L233 L234 | L235 L236 L237 L238 bodies 2 makes body 4 at (45.3177, -46.5494, 36.3293) makes body 5 at (37.0807, -46.0262, 36.1454) makes body 6 at (-4.9607, -45.8781, 36.2935) makes body 7 at (43.3666, -47.1631, 36.4227) makes body 8 at (-6.5096, -46.3993, 35.7723) in component "BOX"
sketch "Sketch23" plane through (0, 0, 55) normal (0, 0, 1) x (-1, 0, 0) in component "BOX"
  line L0 (65, 30) -> (-65, 30)
  line L1 (-65, 30) -> (-65, -60)
  line L2 (-65, -60) -> (65, -60)
  line L3 (65, -60) -> (65, 30)
  line L4 (56.8223, 1.6907) -> (56.8223, -8.0112)
  line L5 (56.8223, -8.0112) -> (60.4465, -8.0112)
  line L6 (60.4465, -8.0112) -> (60.4465, -9.3093)
  line L7 (60.4465, -9.3093) -> (51.7275, -9.3093)
  line L8 (51.7275, -9.3093) -> (51.7275, -8.0112)
  line L9 (51.7275, -8.0112) -> (55.3667, -8.0112)
  line L10 (55.3667, -8.0112) -> (55.3667, 1.6907)
  line L11 (55.3667, 1.6907) -> (56.8223, 1.6907)
  line L12 (50.2043, 1.6907) -> (50.2043, -9.3093)
  line L13 (50.2043, -9.3093) -> (42.2507, -9.3093)
  line L14 (42.2507, -9.3093) -> (42.2507, -8.0112)
  line L15 (42.2507, -8.0112) -> (48.7487, -8.0112)
  line L16 (48.7487, -8.0112) -> (48.7487, -4.6422)
  line L17 (48.7487, -4.6422) -> (42.6634, -4.6422)
  line L18 (42.6634, -4.6422) -> (42.6634, -3.3516)
  line L19 (42.6634, -3.3516) -> (48.7487, -3.3516)
  line L20 (48.7487, -3.3516) -> (48.7487, 0.3926)
  line L21 (48.7487, 0.3926) -> (41.9956, 0.3926)
  line L22 (41.9956, 0.3926) -> (41.9956, 1.6907)
  line L23 (41.9956, 1.6907) -> (50.2043, 1.6907)
  line L24 (32.1361, -2.1661) -> (30.6805, -1.7984)
  spline S0 degree 2 poles (30.6805, -1.7984) (31.1382, -0.0051) (32.3275, 0.9366) knots 0 0 0 1 1 1
  spline S1 degree 2 poles (32.3275, 0.9366) (33.5167, 1.8783) (35.235, 1.8783) knots 0 0 0 1 1 1
  spline S2 degree 2 poles (35.235, 1.8783) (37.0133, 1.8783) (38.1276, 1.1542) knots 0 0 0 1 1 1
  spline S3 degree 2 poles (38.1276, 1.1542) (39.2418, 0.4301) (39.8234, -0.943) knots 0 0 0 1 1 1
  spline S4 degree 2 poles (39.8234, -0.943) (40.4049, -2.3161) (40.4049, -3.8919) knots 0 0 0 1 1 1
  spline S5 degree 2 poles (40.4049, -3.8919) (40.4049, -5.6101) (39.7483, -6.8895) knots 0 0 0 1 1 1
  spline S6 degree 2 poles (39.7483, -6.8895) (39.0918, -8.1688) (37.88, -8.8329) knots 0 0 0 1 1 1
  spline S7 degree 2 poles (37.88, -8.8329) (36.6682, -9.4969) (35.2125, -9.4969) knots 0 0 0 1 1 1
  spline S8 degree 2 poles (35.2125, -9.4969) (33.5618, -9.4969) (32.4363, -8.6565) knots 0 0 0 1 1 1
  spline S9 degree 2 poles (32.4363, -8.6565) (31.3107, -7.8161) (30.868, -6.293) knots 0 0 0 1 1 1
  line L25 (30.868, -6.293) -> (32.3012, -5.9553)
  spline S10 degree 2 poles (32.3012, -5.9553) (32.6839, -7.1558) (33.4117, -7.7036) knots 0 0 0 1 1 1
  spline S11 degree 2 poles (33.4117, -7.7036) (34.1395, -8.2513) (35.2425, -8.2513) knots 0 0 0 1 1 1
  spline S12 degree 2 poles (35.2425, -8.2513) (36.5106, -8.2513) (37.3622, -7.6436) knots 0 0 0 1 1 1
  spline S13 degree 2 poles (37.3622, -7.6436) (38.2139, -7.0358) (38.559, -6.0116) knots 0 0 0 1 1 1
  spline S14 degree 2 poles (38.559, -6.0116) (38.9042, -4.9874) (38.9042, -3.8994) knots 0 0 0 1 1 1
  spline S15 degree 2 poles (38.9042, -3.8994) (38.9042, -2.4962) (38.4953, -1.4495) knots 0 0 0 1 1 1
  spline S16 degree 2 poles (38.4953, -1.4495) (38.0863, -0.4028) (37.2234, 0.115) knots 0 0 0 1 1 1
  spline S17 degree 2 poles (37.2234, 0.115) (36.3605, 0.6327) (35.3551, 0.6327) knots 0 0 0 1 1 1
  spline S18 degree 2 poles (35.3551, 0.6327) (34.132, 0.6327) (33.2841, -0.0726) knots 0 0 0 1 1 1
  spline S19 degree 2 poles (33.2841, -0.0726) (32.4363, -0.7779) (32.1361, -2.1661) knots 0 0 0 1 1 1
  line L26 (28.8421, 1.6907) -> (28.8421, -9.3093)
  line L27 (28.8421, -9.3093) -> (27.3865, -9.3093)
  line L28 (27.3865, -9.3093) -> (27.3865, -4.7923)
  line L29 (27.3865, -4.7923) -> (21.6689, -4.7923)
  line L30 (21.6689, -4.7923) -> (21.6689, -9.3093)
  line L31 (21.6689, -9.3093) -> (20.2132, -9.3093)
  line L32 (20.2132, -9.3093) -> (20.2132, 1.6907)
  line L33 (20.2132, 1.6907) -> (21.6689, 1.6907)
  line L34 (21.6689, 1.6907) -> (21.6689, -3.4942)
  line L35 (21.6689, -3.4942) -> (27.3865, -3.4942)
  line L36 (27.3865, -3.4942) -> (27.3865, 1.6907)
  line L37 (27.3865, 1.6907) -> (28.8421, 1.6907)
  line L38 (17.8046, 1.6907) -> (17.8046, -9.3093)
  line L39 (17.8046, -9.3093) -> (16.3114, -9.3093)
  line L40 (16.3114, -9.3093) -> (10.5338, -0.6729)
  line L41 (10.5338, -0.6729) -> (10.5338, -9.3093)
  line L42 (10.5338, -9.3093) -> (9.1382, -9.3093)
  line L43 (9.1382, -9.3093) -> (9.1382, 1.6907)
  line L44 (9.1382, 1.6907) -> (10.6313, 1.6907)
  line L45 (10.6313, 1.6907) -> (16.409, -6.9533)
  line L46 (16.409, -6.9533) -> (16.409, 1.6907)
  line L47 (16.409, 1.6907) -> (17.8046, 1.6907)
  spline S20 degree 2 poles (7.1348, -3.6668) (7.1348, -6.4055) (5.6641, -7.955) knots 0 0 0 1 1 1
  spline S21 degree 2 poles (5.6641, -7.955) (4.1934, -9.5044) (1.8674, -9.5044) knots 0 0 0 1 1 1
  spline S22 degree 2 poles (1.8674, -9.5044) (0.3442, -9.5044) (-0.8789, -8.7766) knots 0 0 0 1 1 1
  spline S23 degree 2 poles (-0.8789, -8.7766) (-2.1019, -8.0488) (-2.7435, -6.7469) knots 0 0 0 1 1 1
  spline S24 degree 2 poles (-2.7435, -6.7469) (-3.385, -5.4451) (-3.385, -3.7943) knots 0 0 0 1 1 1
  spline S25 degree 2 poles (-3.385, -3.7943) (-3.385, -2.1211) (-2.7097, -0.8005) knots 0 0 0 1 1 1
  spline S26 degree 2 poles (-2.7097, -0.8005) (-2.0344, 0.5201) (-0.7964, 1.1992) knots 0 0 0 1 1 1
  spline S27 degree 2 poles (-0.7964, 1.1992) (0.4417, 1.8783) (1.8749, 1.8783) knots 0 0 0 1 1 1
  spline S28 degree 2 poles (1.8749, 1.8783) (3.4281, 1.8783) (4.6511, 1.1279) knots 0 0 0 1 1 1
  spline S29 degree 2 poles (4.6511, 1.1279) (5.8742, 0.3776) (6.5045, -0.9205) knots 0 0 0 1 1 1
  spline S30 degree 2 poles (6.5045, -0.9205) (7.1348, -2.2186) (7.1348, -3.6668) knots 0 0 0 1 1 1
  spline S31 degree 2 poles (5.6341, -3.6443) (5.6341, -1.6558) (4.5648, -0.5116) knots 0 0 0 1 1 1
  spline S32 degree 2 poles (4.5648, -0.5116) (3.4956, 0.6327) (1.8824, 0.6327) knots 0 0 0 1 1 1
  spline S33 degree 2 poles (1.8824, 0.6327) (0.2391, 0.6327) (-0.8226, -0.5228) knots 0 0 0 1 1 1
  spline S34 degree 2 poles (-0.8226, -0.5228) (-1.8843, -1.6784) (-1.8843, -3.8018) knots 0 0 0 1 1 1
  spline S35 degree 2 poles (-1.8843, -3.8018) (-1.8843, -5.1449) (-1.4304, -6.1466) knots 0 0 0 1 1 1
  spline S36 degree 2 poles (-1.4304, -6.1466) (-0.9764, -7.1483) (-0.1023, -7.6998) knots 0 0 0 1 1 1
  spline S37 degree 2 poles (-0.1023, -7.6998) (0.7719, -8.2513) (1.8599, -8.2513) knots 0 0 0 1 1 1
  spline S38 degree 2 poles (1.8599, -8.2513) (3.4056, -8.2513) (4.5198, -7.1896) knots 0 0 0 1 1 1
  spline S39 degree 2 poles (4.5198, -7.1896) (5.6341, -6.1279) (5.6341, -3.6443) knots 0 0 0 1 1 1
  line L48 (-5.2009, 1.6907) -> (-5.2009, -9.3093)
  line L49 (-5.2009, -9.3093) -> (-6.6565, -9.3093)
  line L50 (-6.6565, -9.3093) -> (-6.6565, 0.3926)
  line L51 (-6.6565, 0.3926) -> (-12.074, 0.3926)
  line L52 (-12.074, 0.3926) -> (-12.074, 1.6907)
  line L53 (-12.074, 1.6907) -> (-5.2009, 1.6907)
  spline S40 degree 2 poles (-13.3646, -3.6668) (-13.3646, -6.4055) (-14.8352, -7.955) knots 0 0 0 1 1 1
  spline S41 degree 2 poles (-14.8352, -7.955) (-16.3059, -9.5044) (-18.632, -9.5044) knots 0 0 0 1 1 1
  spline S42 degree 2 poles (-18.632, -9.5044) (-20.1551, -9.5044) (-21.3782, -8.7766) knots 0 0 0 1 1 1
  spline S43 degree 2 poles (-21.3782, -8.7766) (-22.6013, -8.0488) (-23.2428, -6.7469) knots 0 0 0 1 1 1
  spline S44 degree 2 poles (-23.2428, -6.7469) (-23.8844, -5.4451) (-23.8844, -3.7943) knots 0 0 0 1 1 1
  spline S45 degree 2 poles (-23.8844, -3.7943) (-23.8844, -2.1211) (-23.209, -0.8005) knots 0 0 0 1 1 1
  spline S46 degree 2 poles (-23.209, -0.8005) (-22.5337, 0.5201) (-21.2957, 1.1992) knots 0 0 0 1 1 1
  spline S47 degree 2 poles (-21.2957, 1.1992) (-20.0576, 1.8783) (-18.6245, 1.8783) knots 0 0 0 1 1 1
  spline S48 degree 2 poles (-18.6245, 1.8783) (-17.0712, 1.8783) (-15.8482, 1.1279) knots 0 0 0 1 1 1
  spline S49 degree 2 poles (-15.8482, 1.1279) (-14.6251, 0.3776) (-13.9949, -0.9205) knots 0 0 0 1 1 1
  spline S50 degree 2 poles (-13.9949, -0.9205) (-13.3646, -2.2186) (-13.3646, -3.6668) knots 0 0 0 1 1 1
  spline S51 degree 2 poles (-14.8652, -3.6443) (-14.8652, -1.6558) (-15.9345, -0.5116) knots 0 0 0 1 1 1
  spline S52 degree 2 poles (-15.9345, -0.5116) (-17.0037, 0.6327) (-18.6169, 0.6327) knots 0 0 0 1 1 1
  spline S53 degree 2 poles (-18.6169, 0.6327) (-20.2602, 0.6327) (-21.3219, -0.5228) knots 0 0 0 1 1 1
  spline S54 degree 2 poles (-21.3219, -0.5228) (-22.3837, -1.6784) (-22.3837, -3.8018) knots 0 0 0 1 1 1
  spline S55 degree 2 poles (-22.3837, -3.8018) (-22.3837, -5.1449) (-21.9297, -6.1466) knots 0 0 0 1 1 1
  spline S56 degree 2 poles (-21.9297, -6.1466) (-21.4758, -7.1483) (-20.6016, -7.6998) knots 0 0 0 1 1 1
  spline S57 degree 2 poles (-20.6016, -7.6998) (-19.7275, -8.2513) (-18.6395, -8.2513) knots 0 0 0 1 1 1
  spline S58 degree 2 poles (-18.6395, -8.2513) (-17.0938, -8.2513) (-15.9795, -7.1896) knots 0 0 0 1 1 1
  spline S59 degree 2 poles (-15.9795, -7.1896) (-14.8652, -6.1279) (-14.8652, -3.6443) knots 0 0 0 1 1 1
  line L54 (-30.9075, -2.6238) -> (-30.9075, -3.9144)
  line L55 (-30.9075, -3.9144) -> (-35.5672, -3.9219)
  line L56 (-35.5672, -3.9219) -> (-35.5672, 0.16)
  spline S60 degree 2 poles (-35.5672, 0.16) (-34.4942, 1.0154) (-33.3537, 1.4468) knots 0 0 0 1 1 1
  spline S61 degree 2 poles (-33.3537, 1.4468) (-32.2131, 1.8783) (-31.0126, 1.8783) knots 0 0 0 1 1 1
  spline S62 degree 2 poles (-31.0126, 1.8783) (-29.3919, 1.8783) (-28.0675, 1.1842) knots 0 0 0 1 1 1
  spline S63 degree 2 poles (-28.0675, 1.1842) (-26.7431, 0.4901) (-26.0678, -0.823) knots 0 0 0 1 1 1
  spline S64 degree 2 poles (-26.0678, -0.823) (-25.3925, -2.1361) (-25.3925, -3.7568) knots 0 0 0 1 1 1
  spline S65 degree 2 poles (-25.3925, -3.7568) (-25.3925, -5.3625) (-26.0641, -6.7544) knots 0 0 0 1 1 1
  spline S66 degree 2 poles (-26.0641, -6.7544) (-26.7356, -8.1463) (-27.9962, -8.8216) knots 0 0 0 1 1 1
  spline S67 degree 2 poles (-27.9962, -8.8216) (-29.2568, -9.4969) (-30.9, -9.4969) knots 0 0 0 1 1 1
  spline S68 degree 2 poles (-30.9, -9.4969) (-32.0931, -9.4969) (-33.0573, -9.1105) knots 0 0 0 1 1 1
  spline S69 degree 2 poles (-33.0573, -9.1105) (-34.0215, -8.7241) (-34.5692, -8.0337) knots 0 0 0 1 1 1
  spline S70 degree 2 poles (-34.5692, -8.0337) (-35.117, -7.3434) (-35.4021, -6.2329) knots 0 0 0 1 1 1
  line L57 (-35.4021, -6.2329) -> (-34.089, -5.8728)
  spline S71 degree 2 poles (-34.089, -5.8728) (-33.8414, -6.7131) (-33.4737, -7.1934) knots 0 0 0 1 1 1
  spline S72 degree 2 poles (-33.4737, -7.1934) (-33.106, -7.6736) (-32.4232, -7.9625) knots 0 0 0 1 1 1
  spline S73 degree 2 poles (-32.4232, -7.9625) (-31.7404, -8.2513) (-30.9075, -8.2513) knots 0 0 0 1 1 1
  spline S74 degree 2 poles (-30.9075, -8.2513) (-29.9096, -8.2513) (-29.1818, -7.9475) knots 0 0 0 1 1 1
  spline S75 degree 2 poles (-29.1818, -7.9475) (-28.4539, -7.6436) (-28.0075, -7.1483) knots 0 0 0 1 1 1
  spline S76 degree 2 poles (-28.0075, -7.1483) (-27.561, -6.6531) (-27.3134, -6.0603) knots 0 0 0 1 1 1
  spline S77 degree 2 poles (-27.3134, -6.0603) (-26.8932, -5.0399) (-26.8932, -3.8468) knots 0 0 0 1 1 1
  spline S78 degree 2 poles (-26.8932, -3.8468) (-26.8932, -2.3762) (-27.3997, -1.3857) knots 0 0 0 1 1 1
  spline S79 degree 2 poles (-27.3997, -1.3857) (-27.9062, -0.3953) (-28.8741, 0.0849) knots 0 0 0 1 1 1
  spline S80 degree 2 poles (-28.8741, 0.0849) (-29.8421, 0.5652) (-30.9301, 0.5652) knots 0 0 0 1 1 1
  spline S81 degree 2 poles (-30.9301, 0.5652) (-31.8755, 0.5652) (-32.7759, 0.2012) knots 0 0 0 1 1 1
  spline S82 degree 2 poles (-32.7759, 0.2012) (-33.6763, -0.1627) (-34.1415, -0.5754) knots 0 0 0 1 1 1
  line L58 (-34.1415, -0.5754) -> (-34.1415, -2.6238)
  line L59 (-34.1415, -2.6238) -> (-30.9075, -2.6238)
  line L60 (-37.9608, 1.6907) -> (-37.9608, -9.3093)
  line L61 (-37.9608, -9.3093) -> (-39.4164, -9.3093)
  line L62 (-39.4164, -9.3093) -> (-39.4164, 1.6907)
  line L63 (-39.4164, 1.6907) -> (-37.9608, 1.6907)
  line L64 (-42.0126, 1.6907) -> (-42.0126, -9.3093)
  line L65 (-42.0126, -9.3093) -> (-49.9662, -9.3093)
  line L66 (-49.9662, -9.3093) -> (-49.9662, -8.0112)
  line L67 (-49.9662, -8.0112) -> (-43.4682, -8.0112)
  line L68 (-43.4682, -8.0112) -> (-43.4682, -4.6422)
  line L69 (-43.4682, -4.6422) -> (-49.5535, -4.6422)
  line L70 (-49.5535, -4.6422) -> (-49.5535, -3.3516)
  line L71 (-49.5535, -3.3516) -> (-43.4682, -3.3516)
  line L72 (-43.4682, -3.3516) -> (-43.4682, 0.3926)
  line L73 (-43.4682, 0.3926) -> (-50.2213, 0.3926)
  line L74 (-50.2213, 0.3926) -> (-50.2213, 1.6907)
  line L75 (-50.2213, 1.6907) -> (-42.0126, 1.6907)
  line L76 (-51.737, -1.8434) -> (-53.1101, -1.9635)
  spline S83 degree 2 poles (-53.1101, -1.9635) (-53.2077, -1.1381) (-53.5641, -0.6091) knots 0 0 0 1 1 1
  spline S84 degree 2 poles (-53.5641, -0.6091) (-53.9205, -0.0801) (-54.6708, 0.2463) knots 0 0 0 1 1 1
  spline S85 degree 2 poles (-54.6708, 0.2463) (-55.4212, 0.5727) (-56.3591, 0.5727) knots 0 0 0 1 1 1
  spline S86 degree 2 poles (-56.3591, 0.5727) (-57.192, 0.5727) (-57.8298, 0.3251) knots 0 0 0 1 1 1
  spline S87 degree 2 poles (-57.8298, 0.3251) (-58.4676, 0.0774) (-58.779, -0.354) knots 0 0 0 1 1 1
  spline S88 degree 2 poles (-58.779, -0.354) (-59.0904, -0.7855) (-59.0904, -1.2957) knots 0 0 0 1 1 1
  spline S89 degree 2 poles (-59.0904, -1.2957) (-59.0904, -1.8134) (-58.7902, -2.1998) knots 0 0 0 1 1 1
  spline S90 degree 2 poles (-58.7902, -2.1998) (-58.4901, -2.5863) (-57.7998, -2.8489) knots 0 0 0 1 1 1
  spline S91 degree 2 poles (-57.7998, -2.8489) (-57.3571, -3.0215) (-55.8414, -3.3854) knots 0 0 0 1 1 1
  spline S92 degree 2 poles (-55.8414, -3.3854) (-54.3257, -3.7493) (-53.7179, -4.0719) knots 0 0 0 1 1 1
  spline S93 degree 2 poles (-53.7179, -4.0719) (-52.9301, -4.4846) (-52.5436, -5.0962) knots 0 0 0 1 1 1
  spline S94 degree 2 poles (-52.5436, -5.0962) (-52.1572, -5.7077) (-52.1572, -6.4655) knots 0 0 0 1 1 1
  spline S95 degree 2 poles (-52.1572, -6.4655) (-52.1572, -7.2984) (-52.6299, -8.0225) knots 0 0 0 1 1 1
  spline S96 degree 2 poles (-52.6299, -8.0225) (-53.1026, -8.7466) (-54.0105, -9.1217) knots 0 0 0 1 1 1
  spline S97 degree 2 poles (-54.0105, -9.1217) (-54.9185, -9.4969) (-56.029, -9.4969) knots 0 0 0 1 1 1
  spline S98 degree 2 poles (-56.029, -9.4969) (-57.252, -9.4969) (-58.1862, -9.103) knots 0 0 0 1 1 1
  spline S99 degree 2 poles (-58.1862, -9.103) (-59.1204, -8.7091) (-59.6231, -7.9437) knots 0 0 0 1 1 1
  spline S100 degree 2 poles (-59.6231, -7.9437) (-60.1258, -7.1784) (-60.1633, -6.2104) knots 0 0 0 1 1 1
  line L77 (-60.1633, -6.2104) -> (-58.7677, -6.1054)
  spline S101 degree 2 poles (-58.7677, -6.1054) (-58.6552, -7.1483) (-58.0061, -7.6811) knots 0 0 0 1 1 1
  spline S102 degree 2 poles (-58.0061, -7.6811) (-57.3571, -8.2138) (-56.089, -8.2138) knots 0 0 0 1 1 1
  spline S103 degree 2 poles (-56.089, -8.2138) (-54.7684, -8.2138) (-54.1644, -7.7299) knots 0 0 0 1 1 1
  spline S104 degree 2 poles (-54.1644, -7.7299) (-53.5604, -7.2459) (-53.5604, -6.5631) knots 0 0 0 1 1 1
  spline S105 degree 2 poles (-53.5604, -6.5631) (-53.5604, -5.9703) (-53.988, -5.5876) knots 0 0 0 1 1 1
  spline S106 degree 2 poles (-53.988, -5.5876) (-54.4082, -5.205) (-56.1828, -4.8035) knots 0 0 0 1 1 1
  spline S107 degree 2 poles (-56.1828, -4.8035) (-57.9573, -4.4021) (-58.6176, -4.102) knots 0 0 0 1 1 1
  spline S108 degree 2 poles (-58.6176, -4.102) (-59.5781, -3.6593) (-60.0358, -2.9802) knots 0 0 0 1 1 1
  spline S109 degree 2 poles (-60.0358, -2.9802) (-60.4935, -2.3011) (-60.4935, -1.4157) knots 0 0 0 1 1 1
  spline S110 degree 2 poles (-60.4935, -1.4157) (-60.4935, -0.5378) (-59.9908, 0.2388) knots 0 0 0 1 1 1
  spline S111 degree 2 poles (-59.9908, 0.2388) (-59.488, 1.0154) (-58.5464, 1.4468) knots 0 0 0 1 1 1
  spline S112 degree 2 poles (-58.5464, 1.4468) (-57.6047, 1.8783) (-56.4267, 1.8783) knots 0 0 0 1 1 1
  spline S113 degree 2 poles (-56.4267, 1.8783) (-54.9335, 1.8783) (-53.9243, 1.4431) knots 0 0 0 1 1 1
  spline S114 degree 2 poles (-53.9243, 1.4431) (-52.9151, 1.0079) (-52.341, 0.1337) knots 0 0 0 1 1 1
  spline S115 degree 2 poles (-52.341, 0.1337) (-51.767, -0.7404) (-51.737, -1.8434) knots 0 0 0 1 1 1
  line L78 (35.8311, -32.1846) -> (33.9587, -32.3483)
  spline S116 degree 2 poles (33.9587, -32.3483) (33.8257, -31.2228) (33.3396, -30.5015) knots 0 0 0 1 1 1
  spline S117 degree 2 poles (33.3396, -30.5015) (32.8536, -29.7801) (31.8304, -29.335) knots 0 0 0 1 1 1
  spline S118 degree 2 poles (31.8304, -29.335) (30.8072, -28.8899) (29.5282, -28.8899) knots 0 0 0 1 1 1
  spline S119 degree 2 poles (29.5282, -28.8899) (28.3925, -28.8899) (27.5228, -29.2276) knots 0 0 0 1 1 1
  spline S120 degree 2 poles (27.5228, -29.2276) (26.6531, -29.5653) (26.2285, -30.1536) knots 0 0 0 1 1 1
  spline S121 degree 2 poles (26.2285, -30.1536) (25.8038, -30.7419) (25.8038, -31.4377) knots 0 0 0 1 1 1
  spline S122 degree 2 poles (25.8038, -31.4377) (25.8038, -32.1437) (26.2131, -32.6706) knots 0 0 0 1 1 1
  spline S123 degree 2 poles (26.2131, -32.6706) (26.6224, -33.1976) (27.5637, -33.5557) knots 0 0 0 1 1 1
  spline S124 degree 2 poles (27.5637, -33.5557) (28.1674, -33.791) (30.2343, -34.2873) knots 0 0 0 1 1 1
  spline S125 degree 2 poles (30.2343, -34.2873) (32.3011, -34.7835) (33.1299, -35.2235) knots 0 0 0 1 1 1